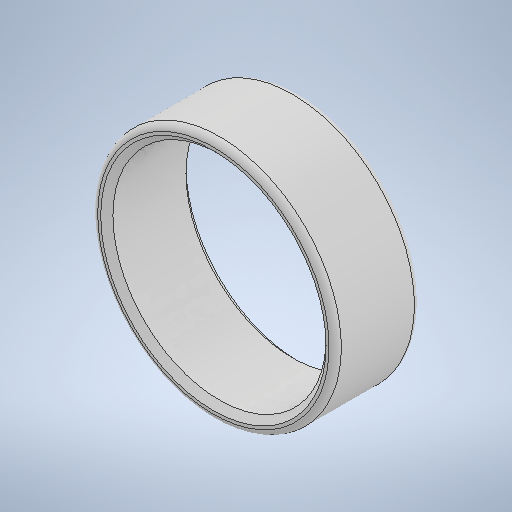
# Autodesk Inventor part: 26-10-206 Spannrad Stufe 2, Riemenspanner
Saved by Autodesk Inventor 2025.2 (Build 292293000, 293)
## iProperties
Created: 2025-01-09
Part Number: 26-10-206 Spannrad Stufe 2, Riemenspanner
Material: Generic
Document SubType Name: Modeling
Designer: Zvonko.Gabric
Density: 1 g/cm^3
Appearance: Default
Author: Zvonko.Gabric
Autodesk Inventor part; units mm, degrees
ref_plane "YZ Plane" through (0, 0, 0) normal (1, 0, 0) x (0, 1, 0)
ref_plane "XZ Plane" through (0, 0, 0) normal (0, 1, 0) x (-1, 0, 0)
ref_plane "XY Plane" through (0, 0, 0) normal (0, 0, 1) x (1, 0, 0)
sketch "Sketch1" plane through (0, 0, 0) normal (0, 1, 0) x (-1, 0, 0)
  line L0 (0, 0) -> (0, -14) construction
  line L1 (18.5, 0) -> (19, 0)
  line L2 (20, -1) -> (20, -13)
  line L3 (19, -14) -> (18.5, -14)
  line L4 (17.5, -13) -> (17.5, -1)
  arc A0 (20, -1) -> (19, 0) centre (19, -1) ccw
  arc A1 (19, -14) -> (20, -13) centre (19, -13) ccw
  line L5 (18.5, 0) -> (17.5, -1)
  line L6 (18.5, -14) -> (17.5, -13)
  dimension "d0" = 14
  dimension "d1" = 17.5
  dimension "d2" = 20
  dimension "d3" = 14
  dimension "d4" = 1
  dimension "d5" = 18.5
  dimension "d6" = 1
  dimension "d7" = 18.5
  dimension "d8" = 1
  constraints: 14 end point, 4 point on circle, 4 tangent, 2 centre point, 2 parallel, 1 equal radius, 1 horizontal, 1 perpendicular, 1 vertical
  measures "d0" distance of L0.start L0.end
  measures "d1" distance between parallel lines of L0 L4
  measures "d2" distance between parallel lines of L0 L2
  measures "d3" distance of L1.start L3.end
  measures "d4" radius of A0
  measures "d5" distance from line of L0 L1.start
  measures "d6" horizontal distance of L4.end L1.start
  measures "d7" distance from line of L0 L3.end
  measures "d8" horizontal distance of L3.end L4.start
revolve "Revolution1" add sketch "Sketch1" angle 360 about axis through (0, 0, 0) along (0, 0, -1)
body "Solid1"
